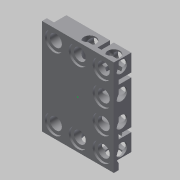
# Autodesk Inventor part: Bumper_front
Saved by Autodesk Inventor 2019.3 (Build 233278000, 278)
## iProperties
Created: 2019-03-06
Part Number: Bumper_front
Material: Generic
Document SubType Name: Modeling
Designer: Varga Daniel
Density: 1 g/cm^3
Appearance: Default
Sheet Metal Rule: Default
Author: Varga Daniel
Autodesk Inventor part; units mm, degrees
ref_plane "YZ Plane" through (0, 0, 0) normal (1, 0, 0) x (0, 1, 0)
ref_plane "XZ Plane" through (0, 0, 0) normal (0, 1, 0) x (-1, 0, 0)
sketch "Sketch7" plane through (0, 0, 0) normal (0, 0, 1) x (1, 0, 0)
  line L0 (5.8, -10.8) -> (5.8, -18)
  line L1 (13.1, -18) -> (5.8, -18)
  line L2 (13.1, -18) -> (13.1, -10.8)
  line L3 (5.8, -10.8) -> (13.1, -10.8)
  circle A0 centre (10, -15) radius 2.5
  line L4 (4.2, -18) -> (4.2, -10.8)
  line L5 (-5, -10.8) -> (4.2, -10.8)
  line L6 (-12, -11.15) -> (-7.6, -11.15)
  line L7 (-14, -11.15) -> (-12, -11.15)
  line L8 (-14, -18) -> (-14, -11.15)
  line L9 (4.2, -18) -> (-14, -18)
  circle A1 centre (0, -15) radius 2.5
  circle A2 centre (-10, -15) radius 2.5
  line L10 (5.8, 18) -> (5.8, 10.8)
  line L11 (13.1, 10.8) -> (5.8, 10.8)
  line L12 (13.1, 18) -> (13.1, 10.8)
  line L13 (5.8, 18) -> (13.1, 18)
  circle A3 centre (10, 15) radius 2.5
  circle A4 centre (-10, 15) radius 2.5
  circle A5 centre (0, 15) radius 2.5
  line L14 (4.2, 10.8) -> (4.2, 18)
  line L15 (-14, 18) -> (4.2, 18)
  line L16 (-14, 11.15) -> (-14, 18)
  line L17 (-12, 11.15) -> (-14, 11.15)
  line L18 (-7.6, 11.15) -> (-12, 11.15)
  line L19 (4.2, 10.8) -> (-5, 10.8)
  line L20 (-15, -9.6) -> (-15, -20)
  line L21 (-15, 20) -> (-15, 9.6)
  line L22 (-15, 9.6) -> (-12, 9.6)
  line L23 (-12, 11.15) -> (-12, 9.6)
  line L24 (-14, 11.15) -> (-12, 11.15)
  line L25 (-14, 11.15) -> (-14, 18)
  line L26 (-14, 18) -> (13.1, 18)
  line L27 (13.1, 18) -> (13.1, -18)
  line L28 (13.1, -18) -> (-14, -18)
  line L29 (-14, -18) -> (-14, -11.15)
  line L30 (-12, -11.15) -> (-14, -11.15)
  line L31 (-12, -9.6) -> (-12, -11.15)
  line L32 (-15, -9.6) -> (-12, -9.6)
  circle A6 centre (0, -15) radius 3.85
  circle A7 centre (10, -15) radius 3.85
  circle A8 centre (10, 15) radius 3.85
  circle A9 centre (0, 15) radius 3.85
  line L33 (-15, -20) -> (-15, 20)
  line L34 (-15, 20) -> (15, 20)
  line L35 (15, 20) -> (15, -20)
  line L36 (15, -20) -> (-15, -20)
  line L37 (-2.086, 7.847) -> (-2.086, -7.847)
  line L38 (-2.086, -7.847) -> (13.1, -7.847)
  line L39 (13.1, -7.847) -> (13.1, 7.847)
  line L40 (13.1, 7.847) -> (-2.086, 7.847)
  circle A10 centre (-10, 15) radius 3.85
  circle A11 centre (-10, -15) radius 3.85
  line L41 (-15, -20) -> (-2.413, -20)
  line L42 (15, 17.413) -> (15, 20)
  line L43 (-2.413, 20) -> (-15, 20)
  line L44 (12.413, 20) -> (12.413, 19.2)
  line L45 (12.413, 19.2) -> (7.587, 19.2)
  line L46 (7.587, 19.2) -> (7.587, 20)
  line L47 (7.587, 20) -> (2.413, 20)
  line L48 (2.413, 20) -> (2.413, 19.2)
  line L49 (2.413, 19.2) -> (-2.413, 19.2)
  line L50 (-2.413, 19.2) -> (-2.413, 20)
  line L51 (15, 20) -> (12.413, 20)
  line L52 (2.413, -19.2) -> (2.413, -20)
  line L53 (7.587, -20) -> (7.587, -19.2)
  line L54 (7.587, -19.2) -> (12.413, -19.2)
  line L55 (12.413, -19.2) -> (12.413, -20)
  line L56 (12.413, -20) -> (15, -20)
  line L57 (-2.413, -20) -> (-2.413, -19.2)
  line L58 (-2.413, -19.2) -> (2.413, -19.2)
  line L59 (14.2, -12.587) -> (15, -12.587)
  line L60 (15, -12.587) -> (15, -7.413)
  line L61 (15, -7.413) -> (14.2, -7.413)
  line L62 (14.2, -7.413) -> (14.2, -2.587)
  line L63 (14.2, -2.587) -> (15, -2.587)
  line L64 (15, -2.587) -> (15, 2.587)
  line L65 (15, 2.587) -> (14.2, 2.587)
  line L66 (14.2, 2.587) -> (14.2, 7.413)
  line L67 (14.2, 7.413) -> (15, 7.413)
  line L68 (15, 7.413) -> (15, 12.587)
  line L69 (15, 12.587) -> (14.2, 12.587)
  line L70 (14.2, 12.587) -> (14.2, 17.413)
  line L71 (14.2, 17.413) -> (15, 17.413)
  line L72 (15, -20) -> (15, -17.413)
  line L73 (15, -17.413) -> (14.2, -17.413)
  line L74 (14.2, -17.413) -> (14.2, -12.587)
  line L75 (2.413, -20) -> (7.587, -20)
  line L76 (-5, -10.8) -> (-5, -6.2)
  line L77 (-7.6, -6.2) -> (-5, -6.2)
  line L78 (-7.6, -6.2) -> (-7.6, -11.15)
  line L79 (-7.6, 6.2) -> (-7.6, 11.15)
  line L80 (-5, 6.2) -> (-7.6, 6.2)
  line L81 (-5, 6.2) -> (-5, 10.8)
  point P0 (0, 0)
  point P1 (-5, -9.6)
  point P2 (-7.6, -9.6)
  point P3 (-7.6, 9.6)
  point P4 (-5, 9.6)
  dimension "d25" = 5
  dimension "d26" = 7.7
  constraints: 162 end point, 12 centre point, 3 other
  measures "d25" diameter of A2
  measures "d26" diameter of A11
extrude "Extrusion6" add sketch "Sketch7" against normal blind 2 contours L3 L2 A7 L1 L0 | L0 L28 L4 L5 L76 L77 L78 L6 L31 L32 L33 L22 L23 L18 L79 L80 L81 L19 L14 L26 L10 L11 L27 L40 L37 L38 L3 | L1 A7 L2 L27 L12 A8 L13 L26 L15 A9 A10 L16 L17 L23 L22 L21 L34 L50 L49 L48 L46 L45 L44 L35 L71 L70 L69 L67 L66 L65 L63 L62 L61 L59 L74 L73 L36 L55 L54 L53 L52 L58 L57 L20 L32 L31 L7 L8 L9 A11 A6 L28 | A7 L2 L1 | L1 A7 | L9 A6 A11 L6 L78 L77 L76 L5 L4 | A7 L2 | L38 L37 L40 L27 | A7 L2 L1 | A6 L9 | L9 A6 | L11 L10 L13 A8 L12 | A11 L9 | L9 A11 | A8 L13 L12 | L12 A8 | L9 L8 L7 L6 A11 | A8 L13 L12 | A8 L13 | L14 L19 L81 L80 L79 L18 A10 L15 A9 | A9 L15 | L15 A9 | A10 L15 | L15 A10 | A10 L18 L17 L16 L15
sketch "Sketch8" plane through (0, 0, 0) normal (0, 0, 1) x (1, 0, 0)
  point P0 (0, 0)
sketch "Sketch9" plane through (0, 0, 0) normal (0, 0, 1) x (1, 0, 0)
  circle A0 centre (0, -15) radius 3.85
  circle A1 centre (10, -15) radius 3.85
  circle A2 centre (10, 15) radius 3.85
  circle A3 centre (0, 15) radius 3.85
  line L0 (-15, -20) -> (-15, 20)
  line L1 (-15, 20) -> (15, 20)
  line L2 (15, 20) -> (15, -20)
  line L3 (15, -20) -> (-15, -20)
  line L4 (-2.086, 7.847) -> (-2.086, -7.847)
  line L5 (-2.086, -7.847) -> (13.1, -7.847)
  line L6 (13.1, -7.847) -> (13.1, 7.847)
  line L7 (13.1, 7.847) -> (-2.086, 7.847)
  circle A4 centre (-10, 15) radius 3.85
  circle A5 centre (-10, -15) radius 3.85
  point P0 (0, 0)
  constraints: 16 end point, 6 centre point
extrude "Extrusion7" cut sketch "Sketch9" against normal blind 0.8 contours A0 | A1 | A2 | A3 | A4 | A5
sketch "Sketch10" plane through (0, 0, -2) normal (0, 0, -1) x (-1, 0, 0)
  line L0 (-5.8, 18) -> (-5.8, 10.8)
  line L1 (-13.1, 10.8) -> (-5.8, 10.8)
  line L2 (-13.1, 18) -> (-13.1, 10.8)
  line L3 (-5.8, 18) -> (-13.1, 18)
  circle A0 centre (-10, 15) radius 2.5
  circle A1 centre (10, 15) radius 2.5
  circle A2 centre (0, 15) radius 2.5
  line L4 (-4.2, 10.8) -> (-4.2, 18)
  line L5 (14, 18) -> (-4.2, 18)
  line L6 (14, 11.15) -> (14, 18)
  line L7 (12, 11.15) -> (14, 11.15)
  line L8 (7.6, 11.15) -> (12, 11.15)
  line L9 (-4.2, 10.8) -> (5, 10.8)
  line L10 (-5.8, -10.8) -> (-5.8, -18)
  line L11 (-13.1, -18) -> (-5.8, -18)
  line L12 (-13.1, -18) -> (-13.1, -10.8)
  line L13 (-5.8, -10.8) -> (-13.1, -10.8)
  circle A3 centre (-10, -15) radius 2.5
  line L14 (-4.2, -18) -> (-4.2, -10.8)
  line L15 (5, -10.8) -> (-4.2, -10.8)
  line L16 (12, -11.15) -> (7.6, -11.15)
  line L17 (14, -11.15) -> (12, -11.15)
  line L18 (14, -18) -> (14, -11.15)
  line L19 (-4.2, -18) -> (14, -18)
  circle A4 centre (0, -15) radius 2.5
  circle A5 centre (10, -15) radius 2.5
  line L20 (14, -11.15) -> (5, -11.15)
  line L21 (5, -11.15) -> (5, -10.8)
  line L22 (5, -10.8) -> (14, -10.8)
  line L23 (14, -10.8) -> (14, -11.15)
  line L24 (5, 10.8) -> (14, 10.8)
  line L25 (14, 10.8) -> (14, 11.15)
  line L26 (14, 11.15) -> (5, 11.15)
  line L27 (5, 11.15) -> (5, 10.8)
  line L28 (7.6, 6.2) -> (7.6, 11.15)
  line L29 (5, 6.2) -> (7.6, 6.2)
  line L30 (5, 6.2) -> (5, 10.8)
  line L31 (5, -10.8) -> (5, -6.2)
  line L32 (7.6, -6.2) -> (5, -6.2)
  line L33 (7.6, -6.2) -> (7.6, -11.15)
  point P0 (0, 0)
  point P1 (7.6, 9.6)
  point P2 (5, 9.6)
  point P3 (5, -9.6)
  point P4 (7.6, -9.6)
  constraints: 68 end point, 6 centre point, 4 parallel, 2 horizontal, 2 perpendicular
extrude "Extrusion8" add sketch "Sketch10" along normal blind 7.2 contours L0 L1 L2 L3 | L4 L5 L6 L7 L8 L26 L27 L9 | L27 L26 L28 L24 | L28 L8 L7 L25 L24 | L10 L11 L12 L13 | L14 L15 L21 L20 L16 L17 L18 L19 | L22 L33 L20 L21 | L17 L16 L33 L22 L23
sketch "Sketch11" plane through (-14, 18, -2) normal (0, 1, 0) x (1, 0, 0)
  circle A0 centre (14, 3) radius 2.5
  circle A1 centre (24, 3) radius 2.5
  line L0 (11.587, -2) -> (-1, -2) construction
  line L1 (-1, 0) -> (11.587, 0) construction
  line L2 (-1, -2) -> (-1, 0) construction
  line L3 (11.587, -2) -> (11.587, 0) projected
  point P0 (14, -2)
  dimension "d24" = 5
  dimension "d27" = 5
  dimension "d29" = 10
  dimension "d30" = 5
  dimension "d31" = 5
  constraints: 2 centre point
  measures "d24" diameter of A0
  measures "d27" diameter of A1
  measures "d29" distance of A0.centre A1.centre
  measures "d30" distance from line of A0.centre L0
  measures "d31" distance from line of A1.centre L0
extrude "Extrusion9" cut sketch "Sketch11" against normal through all
sketch "Sketch12" plane through (13.1, 10.8, -2) normal (1, 0, 0) x (0, 0, -1)
  circle A0 centre (3, 4.2) radius 2.5
  circle A1 centre (3, -25.8) radius 2.5
  line L0 (-2, 6.613) -> (-2, 9.2) construction
  line L1 (0, 9.2) -> (0, 6.613) construction
  line L2 (-2, 9.2) -> (0, 9.2) construction
  line L3 (-2, 6.613) -> (0, 6.613) projected
  point P0 (-2, -10.8)
  dimension "d34" = 5
  dimension "d35" = 5
  dimension "d36" = 5
  dimension "d37" = 5
  dimension "d38" = 5
  constraints: 2 centre point
  measures "d34" diameter of A1
  measures "d35" diameter of A0
  measures "d36" distance from line of A0.centre L2
  measures "d37" distance from line of A0.centre L0
  measures "d38" distance from line of A1.centre L0
extrude "Extrusion10" cut sketch "Sketch12" against normal up to surface (7.3 mm away)
sketch "Sketch13" plane through (12.413, 20, 0) normal (0, 1, 0) x (1, 0, 0)
  line L0 (-14.826, 0) -> (-27.413, 0) projected
  line L1 (-14.826, 0) -> (-14.826, 2) projected
  line L2 (-27.413, 2) -> (-14.826, 2) projected
  line L3 (-27.413, 0) -> (-27.413, 2) projected
  line L4 (-4.826, 0) -> (-10, 0) projected
  line L5 (-4.826, 0) -> (-4.826, 2) projected
  line L6 (-10, 2) -> (-4.826, 2) projected
  line L7 (-10, 0) -> (-10, 2) projected
  line L8 (2.587, 0) -> (0, 0) projected
  line L9 (2.587, 0) -> (2.587, 2) projected
  line L10 (0, 2) -> (2.587, 2) projected
  line L11 (0, 0) -> (0, 2) projected
  line L12 (-14.826, 0) -> (-14.826, 2) construction
  line L13 (-14.826, 0) -> (-10, 0)
  line L14 (-4.826, 0) -> (-10, 0) construction
  line L15 (-4.826, 0) -> (-4.826, 2) construction
  line L16 (-4.826, 0) -> (0, 0)
  line L17 (-12.413, 0) -> (-12.413, 0.9409) construction
  line L18 (-2.413, 0) -> (-2.413, 5) construction
  arc A0 (-4.826, 2) -> (0, 2) centre (-2.413, 5) ccw
  arc A1 (-14.826, 2) -> (-10, 2) centre (-12.413, 5) ccw
  dimension "d42" = 3.85
  dimension "d43" = 3.85
  constraints: 10 end point, 4 perpendicular, 4 point on circle, 2 centre point, 1 coincident, 1 collinear, 1 midpoint
  measures "d42" radius of A0
  measures "d43" radius of A1
extrude "Extrusion11" add sketch "Sketch13" against normal up to surface (0.8 mm away) contours L1 A1 L7 L13 | L5 A0 L11 L16
sketch "Sketch14" plane through (-15, -20, 0) normal (0, -1, 0) x (1, 0, 0)
  line L0 (30, 0) -> (0, 0) projected
  line L1 (30, 0) -> (30, -2) projected
  line L2 (27.413, -2) -> (30, -2) projected
  arc A0 (27.413, -2) -> (22.587, -2) centre (25, -5) ccw projected
  line L3 (17.413, -2) -> (22.587, -2) projected
  arc A1 (17.413, -2) -> (12.587, -2) centre (15, -5) ccw projected
  line L4 (0, -2) -> (12.587, -2) projected
  line L5 (0, 0) -> (0, -2) projected
  point P0 (15, 0)
extrude "Extrusion12" add sketch "Sketch14" against normal up to surface (0.8 mm away)
sketch "Sketch15" plane through (0, 0, -2) normal (0, 0, -1) x (-1, 0, 0)
  line L0 (-2.413, -19.2) -> (-2.413, -20)
  line L1 (-2.413, -20) -> (-7.587, -20)
  line L2 (-7.587, -20) -> (-7.587, -19.2)
  line L3 (-7.587, -19.2) -> (-12.413, -19.2)
  line L4 (-12.413, -19.2) -> (-12.413, -20)
  line L5 (-12.413, -20) -> (-15, -20)
  line L6 (-15, 17.413) -> (-15, 20)
  line L7 (-15, 20) -> (-12.413, 20)
  line L8 (-12.413, 20) -> (-12.413, 19.2)
  line L9 (-12.413, 19.2) -> (-7.587, 19.2)
  line L10 (-7.587, 19.2) -> (-7.587, 20)
  line L11 (-7.587, 20) -> (-2.413, 20)
  line L12 (-2.413, 20) -> (-2.413, 19.2)
  line L13 (-2.413, 19.2) -> (2.413, 19.2)
  line L14 (2.413, 19.2) -> (2.413, 20)
  line L15 (2.413, 20) -> (15, 20)
  line L16 (15, 20) -> (15, 9.6)
  line L17 (15, 9.6) -> (12, 9.6)
  line L18 (12, 11.15) -> (12, 9.6)
  line L19 (14, 11.15) -> (12, 11.15)
  line L20 (14, 11.15) -> (14, 18)
  line L21 (14, 18) -> (-13.1, 18)
  line L22 (-13.1, 18) -> (-13.1, -18)
  line L23 (-13.1, -18) -> (14, -18)
  line L24 (14, -18) -> (14, -11.15)
  line L25 (12, -11.15) -> (14, -11.15)
  line L26 (12, -9.6) -> (12, -11.15)
  line L27 (15, -9.6) -> (12, -9.6)
  line L28 (15, -9.6) -> (15, -20)
  line L29 (15, -20) -> (2.413, -20)
  line L30 (2.413, -20) -> (2.413, -19.2)
  line L31 (2.413, -19.2) -> (-2.413, -19.2)
  line L32 (-12.413, -19.2) -> (-7.587, -19.2) projected
  line L33 (-7.587, -19.2) -> (-7.587, -20) projected
  line L34 (-7.587, -20) -> (-2.413, -20) projected
  line L35 (-2.413, -20) -> (-2.413, -19.2) projected
  line L36 (-2.413, -19.2) -> (2.413, -19.2) projected
  line L37 (2.413, -19.2) -> (2.413, -20) projected
  line L38 (2.413, -20) -> (15, -20) projected
  line L39 (15, -20) -> (15, 20) projected
  line L40 (15, 20) -> (2.413, 20) projected
  line L41 (2.413, 20) -> (2.413, 19.2) projected
  line L42 (2.413, 19.2) -> (-2.413, 19.2) projected
  line L43 (-2.413, 19.2) -> (-2.413, 20) projected
  line L44 (-2.413, 20) -> (-7.587, 20) projected
  line L45 (-7.587, 20) -> (-7.587, 19.2) projected
  line L46 (-7.587, 19.2) -> (-12.413, 19.2) projected
  line L47 (-12.413, 19.2) -> (-12.413, 20) projected
  line L48 (-12.413, 20) -> (-15, 20) projected
  line L49 (-15, 20) -> (-15, 17.413) projected
  line L50 (-15, -20) -> (-12.413, -20) projected
  line L51 (-12.413, -20) -> (-12.413, -19.2) projected
  line L52 (-4.2, 10.8) -> (-4.2, 18) projected
  line L53 (-4.2, 18) -> (14, 18) projected
  line L54 (14, 18) -> (14, 10.8) projected
  line L55 (14, 10.8) -> (-4.2, 10.8) projected
  line L56 (-5.8, 10.8) -> (-13.1, 10.8) projected
  line L57 (-13.1, 10.8) -> (-13.1, 18) projected
  line L58 (-13.1, 18) -> (-5.8, 18) projected
  line L59 (-5.8, 18) -> (-5.8, 10.8) projected
  line L60 (-5.8, -18) -> (-13.1, -18) projected
  line L61 (-13.1, -18) -> (-13.1, -10.8) projected
  line L62 (-13.1, -10.8) -> (-5.8, -10.8) projected
  line L63 (-5.8, -10.8) -> (-5.8, -18) projected
  line L64 (-4.2, -18) -> (-4.2, -10.8) projected
  line L65 (-4.2, -10.8) -> (14, -10.8) projected
  line L66 (14, -10.8) -> (14, -18) projected
  line L67 (14, -18) -> (-4.2, -18) projected
  line L68 (-13.1, -9) -> (-5.8, -9)
  line L69 (-5.8, -9) -> (-5.8, 9)
  line L70 (-5.8, 9) -> (-13.1, 9)
  line L71 (-13.1, 9) -> (-13.1, -9)
  line L72 (-5.8, 0) -> (-10.0472, 0) construction
  line L73 (-13.1, 0) -> (-10.0736, 0) construction
  line L74 (-15, 17.413) -> (-14.2, 17.413) projected
  line L75 (-14.2, 17.413) -> (-14.2, 12.587) projected
  line L76 (-14.2, 12.587) -> (-15, 12.587) projected
  line L77 (-15, 12.587) -> (-15, 7.413) projected
  line L78 (-15, 7.413) -> (-14.2, 7.413) projected
  line L79 (-14.2, 7.413) -> (-14.2, 2.587) projected
  line L80 (-14.2, 2.587) -> (-15, 2.587) projected
  line L81 (-15, 2.587) -> (-15, -2.587) projected
  line L82 (-15, -2.587) -> (-14.2, -2.587) projected
  line L83 (-14.2, -2.587) -> (-14.2, -7.413) projected
  line L84 (-14.2, -7.413) -> (-15, -7.413) projected
  line L85 (-15, -7.413) -> (-15, -12.587) projected
  line L86 (-15, -12.587) -> (-14.2, -12.587) projected
  line L87 (-14.2, -12.587) -> (-14.2, -17.413) projected
  line L88 (-14.2, -17.413) -> (-15, -17.413) projected
  line L89 (-15, -17.413) -> (-15, -20) projected
  line L90 (-14.2, -12.587) -> (-15, -12.587)
  line L91 (-15, -12.587) -> (-15, -7.413)
  line L92 (-15, -7.413) -> (-14.2, -7.413)
  line L93 (-14.2, -7.413) -> (-14.2, -2.587)
  line L94 (-14.2, -2.587) -> (-15, -2.587)
  line L95 (-15, -2.587) -> (-15, 2.587)
  line L96 (-15, 2.587) -> (-14.2, 2.587)
  line L97 (-14.2, 2.587) -> (-14.2, 7.413)
  line L98 (-14.2, 7.413) -> (-15, 7.413)
  line L99 (-15, 7.413) -> (-15, 12.587)
  line L100 (-15, 12.587) -> (-14.2, 12.587)
  line L101 (-14.2, 12.587) -> (-14.2, 17.413)
  line L102 (-14.2, 17.413) -> (-15, 17.413)
  line L103 (-15, -20) -> (-15, -17.413)
  line L104 (-15, -17.413) -> (-14.2, -17.413)
  line L105 (-14.2, -17.413) -> (-14.2, -12.587)
  point P0 (0, 0)
  dimension "d48" = 18
  constraints: 108 end point, 3 perpendicular, 2 collinear, 2 midpoint, 2 parallel, 1 horizontal, 1 point on line
  measures "d48" distance between parallel lines of L70 L68
extrude "Extrusion13" add sketch "Sketch15" along normal up to surface (7.2 mm away) contours L55 L52 L21 L20 L19 L18 | L18 L19 L54 L55 | L22 L70 L69 L68
sketch "Sketch16" plane through (0, 15, -2) normal (0, 0, 1) x (1, 0, 0)
  circle A0 centre (0, 0) radius 2.5 projected
  circle A1 centre (-10, 0) radius 2.5 projected
  point P0 (0, -15)
extrude "Extrusion14" cut sketch "Sketch16" against normal up to next
sketch "Sketch17" plane through (-14, 18, -2) normal (0, 1, 0) x (1, 0, 0)
  circle A0 centre (14, 3) radius 2.5
  line L0 (29, -2) -> (-1, -2) projected
  line L1 (29, -2) -> (29, 0) projected
  line L2 (26.413, 0) -> (29, 0) projected
  arc A1 (21.587, 0) -> (26.413, 0) centre (24, 3) ccw projected
  line L3 (16.413, 0) -> (21.587, 0) projected
  arc A2 (11.587, 0) -> (16.413, 0) centre (14, 3) ccw projected
  line L4 (-1, 0) -> (11.587, 0) projected
  line L5 (-1, -2) -> (-1, 0) projected
  line L6 (29, -2) -> (-1, -2) projected
  line L7 (29, -2) -> (29, 0) projected
  point P0 (14, -2)
  dimension "d53" = 5
  dimension "d54" = 15
  dimension "d55" = 5
  constraints: 1 centre point
  measures "d53" distance from line of A0.centre L6
  measures "d54" distance from line of A0.centre L7
  measures "d55" diameter of A0
extrude "Extrusion15" cut sketch "Sketch17" against normal up to surface (7.2 mm away) contours A0
sketch "Sketch18" plane through (0, 0, 0) normal (0, 0, 1) x (1, 0, 0)
  line L0 (15, -20) -> (15, -17.413) projected
  line L1 (15, -17.413) -> (14.2, -17.413) projected
  line L2 (14.2, -17.413) -> (14.2, -12.587) projected
  line L3 (14.2, -12.587) -> (15, -12.587) projected
  line L4 (15, -12.587) -> (15, -7.413) projected
  line L5 (15, -7.413) -> (14.2, -7.413) projected
  line L6 (14.2, -7.413) -> (14.2, -2.587) projected
  line L7 (14.2, -2.587) -> (15, -2.587) projected
  line L8 (15, -2.587) -> (15, 2.587) projected
  line L9 (15, 2.587) -> (14.2, 2.587) projected
  line L10 (14.2, 2.587) -> (14.2, 7.413) projected
  line L11 (14.2, 7.413) -> (15, 7.413) projected
  line L12 (15, 7.413) -> (15, 12.587) projected
  line L13 (15, 12.587) -> (14.2, 12.587) projected
  line L14 (14.2, 12.587) -> (14.2, 17.413) projected
  line L15 (14.2, 17.413) -> (15, 17.413) projected
  line L16 (15, 17.413) -> (15, 20) projected
  line L17 (15, 20) -> (-15, 20) projected
  line L18 (-15, 20) -> (-15, -20) projected
  line L19 (-15, -20) -> (15, -20) projected
  circle A0 centre (-10, 15) radius 3.85 projected
  circle A1 centre (10, 15) radius 3.85 projected
  circle A2 centre (0, -15) radius 3.85 projected
  circle A3 centre (10, -15) radius 3.85 projected
  circle A4 centre (0, 15) radius 3.85 projected
  circle A5 centre (-10, -15) radius 3.85 projected
  arc A6 (11.7678, 16.7678) -> (8.2322, 16.7678) centre (10, 15) ccw projected
  circle A7 centre (10, 15) radius 2.5
  circle A8 centre (10, 5) radius 2.5
  circle A9 centre (10, -5) radius 2.5
  point P0 (0, 0)
  point P1 (8.2322, 6.7678)
  point P2 (8.2322, -3.2322)
  dimension "d60" = 10
  constraints: 3 vertical, 1 coincident, 13 other
  measures "d60" distance of point (10, 15) point (10, 5)
extrude "Extrusion16" cut sketch "Sketch18" against normal up to surface (9.2 mm away) contours A8 | A9
sketch "Sketch19" plane through (0, 0, 0) normal (0, 0, 1) x (1, 0, 0)
  circle A0 centre (10, 5) radius 2.5 projected
  circle A1 centre (10, -5) radius 2.5 projected
  line L0 (15, -20) -> (15, -17.413) projected
  line L1 (15, -17.413) -> (14.2, -17.413) projected
  line L2 (14.2, -17.413) -> (14.2, -12.587) projected
  line L3 (14.2, -12.587) -> (15, -12.587) projected
  line L4 (15, -12.587) -> (15, -7.413) projected
  line L5 (15, -7.413) -> (14.2, -7.413) projected
  line L6 (14.2, -7.413) -> (14.2, -2.587) projected
  line L7 (14.2, -2.587) -> (15, -2.587) projected
  line L8 (15, -2.587) -> (15, 2.587) projected
  line L9 (15, 2.587) -> (14.2, 2.587) projected
  line L10 (14.2, 2.587) -> (14.2, 7.413) projected
  line L11 (14.2, 7.413) -> (15, 7.413) projected
  line L12 (15, 7.413) -> (15, 12.587) projected
  line L13 (15, 12.587) -> (14.2, 12.587) projected
  line L14 (14.2, 12.587) -> (14.2, 17.413) projected
  line L15 (14.2, 17.413) -> (15, 17.413) projected
  line L16 (15, 17.413) -> (15, 20) projected
  line L17 (15, 20) -> (-15, 20) projected
  line L18 (-15, 20) -> (-15, -20) projected
  line L19 (-15, -20) -> (15, -20) projected
  circle A2 centre (-10, 15) radius 3.85 projected
  circle A3 centre (10, 15) radius 3.85 projected
  circle A4 centre (0, -15) radius 3.85 projected
  circle A5 centre (10, -15) radius 3.85 projected
  circle A6 centre (0, 15) radius 3.85 projected
  circle A7 centre (-10, -15) radius 3.85 projected
  circle A8 centre (10, 5) radius 3.85
  circle A9 centre (10, -5) radius 3.85
  point P0 (0, 0)
  dimension "d67" = 7.7
  dimension "d68" = 7.7
  constraints: 2 centre point, 2 coincident
  measures "d67" diameter of A8
  measures "d68" diameter of A9
extrude "Extrusion17" cut sketch "Sketch19" against normal blind 0.8 contours A8 | A9
sketch "Sketch20" plane through (15, 7.413, 0) normal (1, 0, 0) x (0, 0, -1)
  line L0 (0, 0) -> (0, 5.174) projected
  line L1 (0, 0) -> (2, 0) projected
  line L2 (2, 5.174) -> (2, 0) projected
  line L3 (0, 5.174) -> (2, 5.174) projected
  line L4 (0, 5.174) -> (0, 10) projected
  line L5 (0, 5.174) -> (2, 5.174) projected
  line L6 (2, 10) -> (2, 5.174) projected
  line L7 (0, 10) -> (2, 10) projected
  line L8 (0, -4.826) -> (0, 0) projected
  line L9 (0, -4.826) -> (2, -4.826) projected
  line L10 (2, 0) -> (2, -4.826) projected
  line L11 (0, 0) -> (2, 0) projected
  line L12 (0, -10) -> (0, -4.826) projected
  line L13 (0, -10) -> (2, -10) projected
  line L14 (2, -4.826) -> (2, -10) projected
  line L15 (0, -4.826) -> (2, -4.826) projected
  line L16 (0, -14.826) -> (0, -10) projected
  line L17 (0, -14.826) -> (2, -14.826) projected
  line L18 (2, -10) -> (2, -14.826) projected
  line L19 (0, -10) -> (2, -10) projected
  line L20 (2, -25.413) -> (2, -18.213) projected
  line L21 (0, -20) -> (0, -14.826) projected
  line L22 (0, -20) -> (2, -20) projected
  line L23 (2, -14.826) -> (2, -20) projected
  line L24 (0, -14.826) -> (2, -14.826) projected
  line L25 (0, -24.826) -> (0, -20) projected
  line L26 (0, -24.826) -> (2, -24.826) projected
  line L27 (2, -20) -> (2, -24.826) projected
  line L28 (0, -20) -> (2, -20) projected
  line L29 (2, -24.826) -> (2, -27.413) projected
  line L30 (0, -24.826) -> (2, -24.826) projected
  line L31 (0, -27.413) -> (0, -24.826) projected
  line L32 (0, -27.413) -> (2, -27.413) projected
  line L33 (0, 10) -> (0, 12.587) projected
  line L34 (0, 10) -> (2, 10) projected
  line L35 (2, 12.587) -> (2, 10) projected
  line L36 (0, 12.587) -> (2, 12.587) projected
  line L37 (0, 5.174) -> (0, 10) construction
  line L38 (0, 7.587) -> (5, 7.587) construction
  line L39 (0, 10) -> (2, 10) projected
  arc A0 (2, 10) -> (2, 5.174) centre (5, 7.587) ccw
  line L40 (2, 10) -> (0, 10)
  line L41 (0, 10) -> (0, 5.174)
  line L42 (0, 5.174) -> (2, 5.174) projected
  line L43 (2, 5.174) -> (0, 5.174)
  line L44 (0, -10) -> (0, -4.826) projected
  line L45 (0, -10) -> (2, -10) projected
  line L46 (2, -10) -> (0, -10)
  line L47 (0, -10) -> (0, -14.826)
  line L48 (0, -14.826) -> (2, -14.826) projected
  line L49 (0, -14.826) -> (2, -14.826)
  line L50 (0, -20) -> (2, -20) projected
  line L51 (2, -20) -> (0, -20)
  line L52 (0, -20) -> (0, -24.826)
  line L53 (2, -24.826) -> (0, -24.826)
  arc A1 (2, -20) -> (2, -24.826) centre (5, -22.413) ccw
  arc A2 (2, -10) -> (2, -14.826) centre (5, -12.413) ccw
  line L54 (0, -12.413) -> (3.2383, -12.413) construction
  line L55 (0, -22.413) -> (1.6929, -22.413) construction
  line L56 (0.8, -26.263) -> (0.8, -18.563) construction
  line L57 (2, 0) -> (0, 0)
  line L58 (0, -4.826) -> (0, 0) projected
  line L59 (0, 0) -> (0, -4.826)
  line L60 (0, -4.826) -> (2, -4.826)
  line L61 (0, -2.413) -> (5.1743, -2.413) construction
  arc A3 (2, 0) -> (2, -4.826) centre (5, -2.413) ccw
  point P0 (0, -7.413)
  dimension "d71" = 3.85
  dimension "d73" = 3.85
  dimension "d74" = 3.85
  dimension "d75" = 3.85
  constraints: 32 end point, 8 collinear, 8 point on circle, 7 perpendicular, 4 centre point, 4 midpoint, 3 point on line, 1 coincident
  measures "d71" radius of A0
  measures "d73" radius of A2
  measures "d74" radius of A1
  measures "d75" radius of A3
extrude "Extrusion18" add sketch "Sketch20" against normal up to surface (0.8 mm away) contours L1 A3 L9 L8 | L4 L7 A0 L3 | L9 L14 L13 L12 | L13 A2 L17 L16 | L22 A1 L26 L25
sketch "Sketch21" plane through (13.1, -9, -2) normal (1, 0, 0) x (0, 0, -1)
  circle A0 centre (3, 14) radius 2.5
  circle A1 centre (3, 4) radius 2.5
  line L0 (0, -8.413) -> (0, -11) projected
  arc A2 (0, -3.587) -> (0, -8.413) centre (3, -6) ccw projected
  line L1 (0, 1.587) -> (0, -3.587) projected
  arc A3 (0, 6.413) -> (0, 1.587) centre (3, 4) ccw projected
  line L2 (0, 11.587) -> (0, 6.413) projected
  arc A4 (0, 16.413) -> (0, 11.587) centre (3, 14) ccw projected
  line L3 (0, 21.587) -> (0, 16.413) projected
  arc A5 (0, 26.413) -> (0, 21.587) centre (3, 24) ccw projected
  line L4 (0, 29) -> (0, 26.413) projected
  line L5 (-2, 29) -> (0, 29) projected
  line L6 (-2, -11) -> (-2, 29) projected
  line L7 (-2, -11) -> (0, -11) projected
  line L8 (-2, -11) -> (0, -11) projected
  point P0 (-2, 9)
  dimension "d78" = 5
  dimension "d79" = 5
  dimension "d80" = 5
  dimension "d81" = 5
  dimension "d82" = 15
  dimension "d83" = 10
  dimension "d84" = 10
  constraints: 2 centre point
  measures "d78" distance from line of L6 A0.centre
  measures "d79" distance from line of L6 A1.centre
  measures "d80" diameter of A0
  measures "d81" diameter of A1
  measures "d82" distance from line of A1.centre L8
  measures "d83" distance of A4.centre A1.centre
  measures "d84" distance of A0.centre A3.centre
extrude "Extrusion19" cut sketch "Sketch21" against normal up to surface (7.3 mm away) contours A0 | A1
sketch "Sketch22" plane through (0, 0, -2) normal (0, 0, -1) x (-1, 0, 0)
  circle A0 centre (-10, 5) radius 2.5 projected
  circle A1 centre (-10, -5) radius 2.5 projected
  line L0 (-5.8, 9) -> (-5.8, -9) projected
  line L1 (-5.8, -9) -> (-13.1, -9) projected
  line L2 (-13.1, -9) -> (-13.1, 9) projected
  line L3 (-13.1, 9) -> (-5.8, 9) projected
  line L4 (-7.587, 19.2) -> (-7.587, 20) projected
  line L5 (-7.587, 20) -> (-2.413, 20) projected
  line L6 (-2.413, 20) -> (-2.413, 19.2) projected
  line L7 (-2.413, 19.2) -> (2.413, 19.2) projected
  line L8 (2.413, 19.2) -> (2.413, 20) projected
  line L9 (2.413, 20) -> (15, 20) projected
  line L10 (15, 20) -> (15, -20) projected
  line L11 (15, -20) -> (2.413, -20) projected
  line L12 (2.413, -20) -> (2.413, -19.2) projected
  line L13 (2.413, -19.2) -> (-2.413, -19.2) projected
  line L14 (-2.413, -19.2) -> (-2.413, -20) projected
  line L15 (-2.413, -20) -> (-7.587, -20) projected
  line L16 (-7.587, -20) -> (-7.587, -19.2) projected
  line L17 (-7.587, -19.2) -> (-12.413, -19.2) projected
  line L18 (-12.413, -19.2) -> (-12.413, -20) projected
  line L19 (-12.413, -20) -> (-15, -20) projected
  line L20 (-15, -20) -> (-15, -17.413) projected
  line L21 (-15, -17.413) -> (-14.2, -17.413) projected
  line L22 (-14.2, -17.413) -> (-14.2, -12.587) projected
  line L23 (-14.2, -12.587) -> (-15, -12.587) projected
  line L24 (-15, -12.587) -> (-15, -7.413) projected
  line L25 (-15, -7.413) -> (-14.2, -7.413) projected
  line L26 (-14.2, -7.413) -> (-14.2, -2.587) projected
  line L27 (-14.2, -2.587) -> (-15, -2.587) projected
  line L28 (-15, -2.587) -> (-15, 2.587) projected
  line L29 (-15, 2.587) -> (-14.2, 2.587) projected
  line L30 (-14.2, 2.587) -> (-14.2, 7.413) projected
  line L31 (-14.2, 7.413) -> (-15, 7.413) projected
  line L32 (-15, 7.413) -> (-15, 12.587) projected
  line L33 (-15, 12.587) -> (-14.2, 12.587) projected
  line L34 (-14.2, 12.587) -> (-14.2, 17.413) projected
  line L35 (-14.2, 17.413) -> (-15, 17.413) projected
  line L36 (-15, 17.413) -> (-15, 20) projected
  line L37 (-15, 20) -> (-12.413, 20) projected
  line L38 (-12.413, 20) -> (-12.413, 19.2) projected
  line L39 (-12.413, 19.2) -> (-7.587, 19.2) projected
  line L40 (-4.2, -18) -> (-4.2, -10.8) projected
  line L41 (-4.2, -10.8) -> (14, -10.8) projected
  line L42 (14, -10.8) -> (14, -18) projected
  line L43 (14, -18) -> (-4.2, -18) projected
  line L44 (-5.8, -18) -> (-13.1, -18) projected
  line L45 (-13.1, -18) -> (-13.1, -10.8) projected
  line L46 (-13.1, -10.8) -> (-5.8, -10.8) projected
  line L47 (-5.8, -10.8) -> (-5.8, -18) projected
  line L48 (-5.8, 10.8) -> (-13.1, 10.8) projected
  line L49 (-13.1, 10.8) -> (-13.1, 18) projected
  line L50 (-13.1, 18) -> (-5.8, 18) projected
  line L51 (-5.8, 18) -> (-5.8, 10.8) projected
  line L52 (-4.2, 10.8) -> (-4.2, 18) projected
  line L53 (-4.2, 18) -> (14, 18) projected
  line L54 (14, 18) -> (14, 10.8) projected
  line L55 (14, 10.8) -> (-4.2, 10.8) projected
  circle A2 centre (10, 15) radius 2.5 projected
  circle A3 centre (0, 15) radius 2.5 projected
  circle A4 centre (10, -15) radius 2.5 projected
  circle A5 centre (0, -15) radius 2.5 projected
  circle A6 centre (-10, 15) radius 2.5 projected
  circle A7 centre (-10, -15) radius 2.5 projected
  line L56 (14, -10.8) -> (15, -10.8)
  line L57 (14, 10.8) -> (15, 10.8)
  line L58 (-14.2, -12.587) -> (-15, -12.587)
  line L59 (-15, -12.587) -> (-15, -7.413)
  line L60 (-15, -7.413) -> (-14.2, -7.413)
  line L61 (-14.2, -7.413) -> (-14.2, -2.587)
  line L62 (-14.2, -2.587) -> (-15, -2.587)
  line L63 (-15, -2.587) -> (-15, 2.587)
  line L64 (-15, 2.587) -> (-14.2, 2.587)
  line L65 (-14.2, 2.587) -> (-14.2, 7.413)
  line L66 (-14.2, 7.413) -> (-15, 7.413)
  line L67 (-15, 7.413) -> (-15, 12.587)
  line L68 (-15, 12.587) -> (-14.2, 12.587)
  line L69 (-14.2, 12.587) -> (-14.2, 17.413)
  line L70 (-14.2, 17.413) -> (-15, 17.413)
  line L71 (-15, 17.413) -> (-15, 20)
  line L72 (-15, 20) -> (-12.413, 20)
  line L73 (-12.413, 20) -> (-12.413, 19.2)
  line L74 (-12.413, 19.2) -> (-7.587, 19.2)
  line L75 (-7.587, 19.2) -> (-7.587, 20)
  line L76 (-7.587, 20) -> (-2.413, 20)
  line L77 (-2.413, 20) -> (-2.413, 19.2)
  line L78 (-2.413, 19.2) -> (2.413, 19.2)
  line L79 (2.413, 19.2) -> (2.413, 20)
  line L80 (2.413, 20) -> (15, 20)
  line L81 (15, 20) -> (15, 9.6)
  line L82 (15, 9.6) -> (12, 9.6)
  line L83 (12, 11.15) -> (12, 9.6)
  line L84 (14, 11.15) -> (12, 11.15)
  line L85 (14, 11.15) -> (14, 18)
  line L86 (14, 18) -> (-13.1, 18)
  line L87 (-13.1, 18) -> (-13.1, -18)
  line L88 (-13.1, -18) -> (14, -18)
  line L89 (14, -18) -> (14, -11.15)
  line L90 (12, -11.15) -> (14, -11.15)
  line L91 (12, -9.6) -> (12, -11.15)
  line L92 (15, -9.6) -> (12, -9.6)
  line L93 (15, -9.6) -> (15, -20)
  line L94 (15, -20) -> (2.413, -20)
  line L95 (2.413, -20) -> (2.413, -19.2)
  line L96 (2.413, -19.2) -> (-2.413, -19.2)
  line L97 (-2.413, -19.2) -> (-2.413, -20)
  line L98 (-2.413, -20) -> (-7.587, -20)
  line L99 (-7.587, -20) -> (-7.587, -19.2)
  line L100 (-7.587, -19.2) -> (-12.413, -19.2)
  line L101 (-12.413, -19.2) -> (-12.413, -20)
  line L102 (-12.413, -20) -> (-15, -20)
  line L103 (-15, -20) -> (-15, -17.413)
  line L104 (-15, -17.413) -> (-14.2, -17.413)
  line L105 (-14.2, -17.413) -> (-14.2, -12.587)
  line L106 (6, -9.5) -> (15, -9.5)
  line L107 (6, 9.5) -> (15, 9.5)
  line L108 (6, -9.5) -> (6, 9.5)
  line L109 (15, -9.5) -> (15, 9.5)
  line L110 (20.5, -9.5) -> (11.9557, -9.5) construction
  line L111 (11.9557, -10.95) -> (11.9557, -9.5) construction
  line L112 (10, -10.95) -> (11.9557, -10.95) construction
  line L113 (10, -10.95) -> (10, 10.95) construction
  line L114 (10, 10.95) -> (11.9557, 10.95) construction
  line L115 (11.9557, 10.95) -> (11.9557, 9.5) construction
  line L116 (11.9557, 9.5) -> (20.5, 9.5) construction
  line L117 (20.5, -9.5) -> (20.5, 9.5) construction
  line L118 (-4.2, -18) -> (-4.2, -10.8)
  line L119 (5, -10.8) -> (-4.2, -10.8)
  line L120 (12, -11.15) -> (7.6, -11.15)
  line L121 (14, -11.15) -> (12, -11.15)
  line L122 (14, -18) -> (14, -11.15)
  line L123 (-4.2, -18) -> (14, -18)
  circle A8 centre (0, -15) radius 2.5
  circle A9 centre (10, -15) radius 2.5
  circle A10 centre (10, 15) radius 2.5
  circle A11 centre (0, 15) radius 2.5
  line L124 (-4.2, 10.8) -> (-4.2, 18)
  line L125 (14, 18) -> (-4.2, 18)
  line L126 (14, 11.15) -> (14, 18)
  line L127 (12, 11.15) -> (14, 11.15)
  line L128 (7.6, 11.15) -> (12, 11.15)
  line L129 (-4.2, 10.8) -> (5, 10.8)
  line L130 (5, -10.8) -> (5, -6.2)
  line L131 (7.6, -6.2) -> (5, -6.2)
  line L132 (7.6, -6.2) -> (7.6, -11.15)
  line L133 (7.6, 6.2) -> (7.6, 11.15)
  line L134 (5, 6.2) -> (7.6, 6.2)
  line L135 (5, 6.2) -> (5, 10.8)
  point P0 (0, 0)
  point P1 (5, -9.6)
  point P2 (7.6, -9.6)
  point P3 (7.6, 9.6)
  point P4 (5, 9.6)
  dimension "d87" = 0.1
  dimension "d88" = 0.1
  dimension "d93" = 9
  constraints: 160 end point, 4 centre point, 4 perpendicular, 4 point on line, 1 parallel
  measures "d87" distance between parallel lines of L107 L82
  measures "d88" distance between parallel lines of L106 L92
  measures "d93" distance between parallel lines of L108 L109
extrude "Extrusion21" add sketch "Sketch22" along normal blind 6.9 contours L133 L134 L108 L107 | L107 L10 L106 L132 L131 L108 L134 L133 | L106 L108 L131 L132
sketch "Sketch23" plane through (0, 0, -8.9) normal (0, 0, -1) x (-1, 0, 0)
  circle A0 centre (10, 15) radius 2.5
  circle A1 centre (0, 15) radius 2.5
  line L0 (-4.2, 10.8) -> (-4.2, 18)
  line L1 (14, 18) -> (-4.2, 18)
  line L2 (14, 11.15) -> (14, 18)
  line L3 (12, 11.15) -> (14, 11.15)
  line L4 (7.6, 11.15) -> (12, 11.15)
  line L5 (-4.2, 10.8) -> (5, 10.8)
  line L6 (-4.2, -18) -> (-4.2, -10.8)
  line L7 (5, -10.8) -> (-4.2, -10.8)
  line L8 (12, -11.15) -> (7.6, -11.15)
  line L9 (14, -11.15) -> (12, -11.15)
  line L10 (14, -18) -> (14, -11.15)
  line L11 (-4.2, -18) -> (14, -18)
  circle A2 centre (0, -15) radius 2.5
  circle A3 centre (10, -15) radius 2.5
  line L12 (6, -9.5) -> (15, -9.5) projected
  line L13 (15, -9.5) -> (15, 9.5) projected
  line L14 (15, 9.5) -> (6, 9.5) projected
  line L15 (6, 9.5) -> (6, -9.5) projected
  line L16 (6, -9.5) -> (7.6, -9.5)
  line L17 (7.6, -9.5) -> (7.6, 9.5)
  line L18 (7.6, 9.5) -> (6, 9.5)
  line L19 (6, 9.5) -> (6, -9.5)
  line L20 (7.6, 6.2) -> (7.6, 11.15)
  line L21 (5, 6.2) -> (7.6, 6.2)
  line L22 (5, 6.2) -> (5, 10.8)
  line L23 (5, -10.8) -> (5, -6.2)
  line L24 (7.6, -6.2) -> (5, -6.2)
  line L25 (7.6, -6.2) -> (7.6, -11.15)
  point P0 (0, 0)
  point P1 (7.6, 9.6)
  point P2 (5, 9.6)
  point P3 (5, -9.6)
  point P4 (7.6, -9.6)
  dimension "d97" = 7.4
  constraints: 44 end point, 4 centre point, 2 parallel, 1 collinear, 1 horizontal, 1 perpendicular
  measures "d97" distance between parallel lines of L13 L17
extrude "Extrusion22" add sketch "Sketch23" along normal blind 1 contours L21 L17 L24 L15 | L15 L14 L17 L21 | L24 L17 L12 L15
sketch "Sketch24" plane through (0, 0, -2) normal (0, 0, -1) x (-1, 0, 0)
  circle A0 centre (-10, 5) radius 2.5 projected
  circle A1 centre (-10, -5) radius 2.5 projected
  line L0 (-5.8, 9) -> (-5.8, -9) projected
  line L1 (-5.8, -9) -> (-13.1, -9) projected
  line L2 (-13.1, -9) -> (-13.1, 9) projected
  line L3 (-13.1, 9) -> (-5.8, 9) projected
  line L4 (-7.587, 19.2) -> (-7.587, 20) projected
  line L5 (-7.587, 20) -> (-2.413, 20) projected
  line L6 (-2.413, 20) -> (-2.413, 19.2) projected
  line L7 (-2.413, 19.2) -> (2.413, 19.2) projected
  line L8 (2.413, 19.2) -> (2.413, 20) projected
  line L9 (2.413, 20) -> (15, 20) projected
  line L10 (15, 20) -> (15, 9.5) projected
  line L11 (6, 9.5) -> (15, 9.5) projected
  line L12 (6, -9.5) -> (6, 9.5) projected
  line L13 (15, -9.5) -> (6, -9.5) projected
  line L14 (15, -9.5) -> (15, -20) projected
  line L15 (15, -20) -> (2.413, -20) projected
  line L16 (2.413, -20) -> (2.413, -19.2) projected
  line L17 (2.413, -19.2) -> (-2.413, -19.2) projected
  line L18 (-2.413, -19.2) -> (-2.413, -20) projected
  line L19 (-2.413, -20) -> (-7.587, -20) projected
  line L20 (-7.587, -20) -> (-7.587, -19.2) projected
  line L21 (-7.587, -19.2) -> (-12.413, -19.2) projected
  line L22 (-12.413, -19.2) -> (-12.413, -20) projected
  line L23 (-12.413, -20) -> (-15, -20) projected
  line L24 (-15, -20) -> (-15, -17.413) projected
  line L25 (-15, -17.413) -> (-14.2, -17.413) projected
  line L26 (-14.2, -17.413) -> (-14.2, -12.587) projected
  line L27 (-14.2, -12.587) -> (-15, -12.587) projected
  line L28 (-15, -12.587) -> (-15, -7.413) projected
  line L29 (-15, -7.413) -> (-14.2, -7.413) projected
  line L30 (-14.2, -7.413) -> (-14.2, -2.587) projected
  line L31 (-14.2, -2.587) -> (-15, -2.587) projected
  line L32 (-15, -2.587) -> (-15, 2.587) projected
  line L33 (-15, 2.587) -> (-14.2, 2.587) projected
  line L34 (-14.2, 2.587) -> (-14.2, 7.413) projected
  line L35 (-14.2, 7.413) -> (-15, 7.413) projected
  line L36 (-15, 7.413) -> (-15, 12.587) projected
  line L37 (-15, 12.587) -> (-14.2, 12.587) projected
  line L38 (-14.2, 12.587) -> (-14.2, 17.413) projected
  line L39 (-14.2, 17.413) -> (-15, 17.413) projected
  line L40 (-15, 17.413) -> (-15, 20) projected
  line L41 (-15, 20) -> (-12.413, 20) projected
  line L42 (-12.413, 20) -> (-12.413, 19.2) projected
  line L43 (-12.413, 19.2) -> (-7.587, 19.2) projected
  line L44 (15, 9.5) -> (15, -9.5) projected
  line L45 (-4.2, -18) -> (-4.2, -10.8) projected
  line L46 (-4.2, -10.8) -> (14, -10.8) projected
  line L47 (14, -10.8) -> (14, -18) projected
  line L48 (14, -18) -> (-4.2, -18) projected
  line L49 (-5.8, -18) -> (-13.1, -18) projected
  line L50 (-13.1, -18) -> (-13.1, -10.8) projected
  line L51 (-13.1, -10.8) -> (-5.8, -10.8) projected
  line L52 (-5.8, -10.8) -> (-5.8, -18) projected
  line L53 (-5.8, 10.8) -> (-13.1, 10.8) projected
  line L54 (-13.1, 10.8) -> (-13.1, 18) projected
  line L55 (-13.1, 18) -> (-5.8, 18) projected
  line L56 (-5.8, 18) -> (-5.8, 10.8) projected
  line L57 (-4.2, 10.8) -> (-4.2, 18) projected
  line L58 (-4.2, 18) -> (14, 18) projected
  line L59 (14, 18) -> (14, 10.8) projected
  line L60 (14, 10.8) -> (-4.2, 10.8) projected
  circle A2 centre (10, 15) radius 2.5 projected
  circle A3 centre (0, 15) radius 2.5 projected
  circle A4 centre (10, -15) radius 2.5 projected
  circle A5 centre (0, -15) radius 2.5 projected
  circle A6 centre (-10, 15) radius 2.5 projected
  circle A7 centre (-10, -15) radius 2.5 projected
  line L61 (-0.046, -4.6355) -> (-0.046, -7.747)
  line L62 (-10.5122, -7.747) -> (-0.046, -7.747)
  line L63 (-10.5122, 7.747) -> (-10.5122, -7.747)
  line L64 (-10.5122, 7.747) -> (-0.046, 7.747)
  line L65 (-0.046, 7.747) -> (-0.046, 4.6355)
  line L66 (-0.046, 4.6355) -> (-2.84, 4.6355)
  line L67 (-2.84, 4.6355) -> (-2.84, -4.6355)
  line L68 (-0.046, -4.6355) -> (-2.84, -4.6355)
  line L69 (-8.859, 4.0005) -> (-7.4951, 4.0005)
  line L70 (-8.859, -4.0005) -> (-8.859, 4.0005)
  line L71 (-7.4951, -4.0005) -> (-8.859, -4.0005)
  line L72 (-7.4951, 4.0005) -> (-7.4951, -4.0005)
  line L73 (-0.046, -4.6355) -> (-0.046, -7.747)
  line L74 (-10.5122, -7.747) -> (-0.046, -7.747)
  line L75 (-10.5122, 7.747) -> (-10.5122, -7.747)
  line L76 (-10.5122, 7.747) -> (-0.046, 7.747)
  line L77 (-0.046, 7.747) -> (-0.046, 4.6355)
  line L78 (-0.046, 4.6355) -> (-2.84, 4.6355)
  line L79 (-2.84, 4.6355) -> (-2.84, -4.6355)
  line L80 (-0.046, -4.6355) -> (-2.84, -4.6355)
  line L81 (-8.859, 4.0005) -> (-7.4951, 4.0005)
  line L82 (-8.859, -4.0005) -> (-8.859, 4.0005)
  line L83 (-7.4951, -4.0005) -> (-8.859, -4.0005)
  line L84 (-7.4951, 4.0005) -> (-7.4951, -4.0005)
  line L85 (-1.2, 7.747) -> (-5.2791, 7.747)
  line L86 (-5.2791, -7.747) -> (-1.2, -7.747)
  line L87 (-1.2, -7.747) -> (-1.2, 7.747)
  line L88 (-4.2, 7.747) -> (-4.2, -7.747)
  point P0 (0, 0)
  dimension "d100" = 3
  constraints: 56 end point, 3 point on line, 2 parallel, 1 collinear, 1 horizontal, 1 midpoint
  measures "d100" distance between parallel lines of L88 L87
ref_plane "Work Plane1" through (0.5363, -7.747, -9.2807) normal (0.2164, 0, 0.9763) x (0.9763, 0, -0.2164)
extrude "Extrusion23" add sketch "Sketch24" along normal up to surface contours L64 L87 L66 L67 L68 L62 L88 | L87 L68 L67 L66 surface through (0.5363, -7.747, -9.2807) normal (0.2164, 0, 0.9763)
equation "\"d24\" = d25"
equation "\"d27\" = d25"
equation "\"d34\" = d27"
equation "\"d35\" = d27"
equation "\"d43\" = d42"
equation "\"d55\" = d25"
equation "\"d68\" = d67"
equation "\"BendRadius\" = Thickness"
equation "\"BendReliefWidth\" = Thickness"
equation "\"BendReliefDepth\" = 0.5 * Thickness"
equation "\"CornerReliefSize\" = 4 * Thickness"
equation "\"MinimumRemnant\" = 2 * Thickness"
equation "\"TransitionRadius\" = BendRadius"
equation "\"JacobiRadiusSize\" = Thickness"
equation "\"GapSize\" = Thickness"
equation "\"Thickness\" = 0.5"
body "Solid2"
